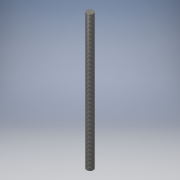
# Autodesk Inventor part: Main Rod
Saved by Autodesk Inventor 2019 (Build 230136000, 136)
## iProperties
Created: 2020-01-30
Part Number: Main Rod
Material: Stainless Steel
Document SubType Name: Modeling
Designer: alb16148
Density: 8 g/cm^3
Appearance: Semi-Polished
Author: alb16148
Autodesk Inventor part; units mm, degrees
ref_plane "YZ Plane" through (0, 0, 0) normal (1, 0, 0) x (0, 1, 0)
ref_plane "XZ Plane" through (0, 0, 0) normal (0, 1, 0) x (-1, 0, 0)
ref_plane "XY Plane" through (0, 0, 0) normal (0, 0, 1) x (1, 0, 0)
sketch "Sketch1" plane through (0, 0, 0) normal (1, 0, 0) x (0, 1, 0)
  line L0 (121, 3) -> (1, 3)
  line L1 (1, 3) -> (1, -3)
  line L2 (1, -3) -> (121, -3)
  line L3 (121, -3) -> (121, 3)
  line L4 (121, 3) -> (1, -3) construction
  line L5 (1, 3) -> (121, -3) construction
  line L6 (10, 8.35) -> (0, 8.35)
  line L7 (0, 8.35) -> (0, 20)
  line L8 (10, 8.35) -> (10, 9.45)
  line L9 (10, 9.45) -> (16, 9.45)
  line L10 (16, 9.45) -> (16, 17)
  line L11 (16, 17) -> (18, 17)
  line L12 (18, 17) -> (18, 18.5)
  line L13 (18, 18.5) -> (16, 18.5)
  line L14 (16, 18.5) -> (16, 20)
  line L15 (16, 20) -> (0, 20)
  line L16 (-24.2, 0) -> (145.2, 0) projected
  line L17 (16, 20) -> (31, 20)
  line L18 (18, 17) -> (31, 17)
  line L19 (75, 9.45) -> (69, 9.45)
  line L20 (69, 9.45) -> (69, 8.35)
  line L21 (69, 8.35) -> (66, 8.35)
  line L22 (75, 9.45) -> (75, 12.45)
  arc A0 (75, 12.45) -> (31, 20) centre (31, -111.9869) ccw
  arc A1 (59.1084, 13.9001) -> (31, 17) centre (31, -111.9869) ccw
  arc A2 (66, 8.35) -> (59.1084, 13.9001) centre (56.9292, 4.1404) ccw
  line L23 (121, 0) -> (1, 0)
  point P0 (0, 0)
  point P1 (61, 0)
  point P2 (61, 0)
  dimension "d0" = 120
  dimension "d1" = 6
  dimension "d5" = 8.35
  dimension "d6" = 9.45
  dimension "d7" = 1.5
  dimension "d8" = 1.5
  dimension "d9" = 20
  dimension "d10" = 6
  dimension "d11" = 2
  dimension "d13" = 10
  dimension "d14" = 1
  dimension "d15" = 6
  dimension "d16" = 3
  dimension "d17" = 9.45
  dimension "d18" = 3
  dimension "d19" = 8.35
  dimension "d20" = 15
  dimension "d21" = 7.55
  dimension "d22" = 75
  dimension "d23" = 10
  constraints: 46 end point, 8 perpendicular, 7 horizontal, 6 point on circle, 5 midpoint, 3 centre point, 3 tangent, 3 vertical, 2 parallel, 2 point on line, 2 vertical alignment, 1 collinear, 1 concentric, 1 horizontal alignment
  measures "d0" distance of L2.end L1.end
  measures "d1" distance of L1.end L0.end
  measures "d5" distance between parallel lines of L16 L6
  measures "d6" distance between parallel lines of L16 L9
  measures "d7" distance between parallel lines of L15 L13
  measures "d8" distance between parallel lines of L13 L11
  measures "d9" distance between parallel lines of L16 L15
  measures "d10" distance of L8.end L9.end
  measures "d11" distance of L12.end L13.end
  measures "d13" distance of L6.start L6.end
  measures "d14" distance from line of point (0, 0) L1
  measures "d15" distance of L19.start L19.end
  measures "d16" distance of L19.start L22.end
  measures "d17" distance between parallel lines of L16 L19
  measures "d18" distance of L20.end L21.end
  measures "d19" distance between parallel lines of L16 L21
  measures "d20" distance of L14.end L17.end
  measures "d21" distance of L9.end L10.end
  measures "d22" distance between parallel lines of L7 L22
  measures "d23" radius of A2
revolve "Revolution1" add sketch "Sketch1" angle 360 about axis through (0, -10, 0) along (0, 1, 0) contours L3 L16 L1 L0
thread "Thread1" size "M6x1" class "6g" standard "ANSI Metric M Profile" full length
body "Solid1"
